Autodesk Fusion 360 part; units mm, degrees
(part 2 of 2)
sketch "All" plane through (0, 0, 0) normal (0, 0, 1) x (1, 0, 0)
  line L0 (911.9011, 0.1672) -> (886.7114, 0.1671)
  line L1 (568.1448, -296.0398) -> (568.1448, -307.8378)
  line L2 (734.5324, -64.7128) -> (810.7324, -64.7128)
  line L3 (909.9675, -283.9081) -> (916.3175, -283.9081)
  line L4 (886.7114, 0.1671) -> (886.7114, 6.5171)
  line L5 (775.9132, -250.6459) -> (775.9132, -244.2911)
  line L6 (662.6478, -251.0469) -> (662.6478, -327.2469)
  line L7 (615.7805, -143.0099) -> (615.7805, -149.3599)
  line L8 (916.3175, -296.6081) -> (909.9675, -296.6081)
  line L9 (861.3114, 6.5171) -> (861.3114, 0.1672)
  line L10 (825.1884, -118.2052) -> (825.181, -105.5052)
  line L11 (848.6114, -82.3828) -> (861.3114, -82.3828)
  line L12 (628.4805, -149.3599) -> (628.4805, -143.0099)
  line L13 (909.9675, -271.2081) -> (909.9675, -244.9009)
  line L14 (732.6938, -144.5054) -> (808.8938, -144.5054)
  line L15 (733.2164, -153.1742) -> (809.4164, -153.1742)
  line L16 (728.1176, -23.0624) -> (728.1101, -10.3624)
  line L17 (916.3175, -309.3081) -> (916.3175, -296.6081)
  line L18 (848.6114, 0.1672) -> (848.6114, 6.5171)
  line L19 (775.9132, -250.6449) -> (744.3131, -250.6449)
  line L20 (914.218, -118.2052) -> (914.2254, -105.5052)
  line L21 (874.0114, 6.5171) -> (874.0114, 0.1672)
  line L22 (561.7948, -307.8378) -> (561.7948, -320.5378)
  line L23 (916.3175, -283.9081) -> (916.3175, -271.2081)
  line L24 (653.8805, -149.3599) -> (666.5805, -149.3599)
  line L25 (817.1471, -23.0624) -> (817.1546, -10.3624)
  line L26 (825.1921, -143.6015) -> (831.6032, -143.6015)
  line L27 (809.4164, -217.5813) -> (809.4164, -232.0956)
  line L28 (732.5584, -251.0469) -> (706.9479, -251.0469)
  line L29 (831.6474, -237.2473) -> (831.6474, -220.0168)
  line L30 (788.6132, -326.8449) -> (814.2237, -326.8449)
  line L31 (827.4175, -271.2081) -> (833.7675, -271.2081)
  line L32 (810.7324, 3.1782) -> (734.4601, 2.7712)
  line L33 (886.7114, -76.0328) -> (886.7114, -82.3828)
  line L34 (628.4805, -143.0099) -> (615.7805, -143.0099)
  line L35 (831.531, -92.3716) -> (831.531, -105.5015)
  line L36 (603.0823, -149.3583) -> (615.7805, -149.3599)
  line L37 (775.9132, -333.1987) -> (788.6132, -333.1987)
  line L38 (568.3687, -250.951) -> (644.5687, -250.951)
  line L39 (568.1448, -296.0398) -> (644.3448, -296.0398)
  line L40 (561.7948, -320.5378) -> (568.1448, -320.5378)
  line L41 (861.3114, -82.3828) -> (861.3114, -76.0328)
  line L42 (706.9479, -327.2469) -> (732.5584, -327.2469)
  line L43 (815.249, -114.5749) -> (815.249, -127.2749)
  line L44 (644.5687, -287.2419) -> (568.3687, -287.2419)
  line L45 (679.2805, -231.9067) -> (666.5805, -231.9067)
  line L46 (815.249, -127.2749) -> (808.8937, -127.2749)
  line L47 (833.7675, -283.9081) -> (833.7675, -296.6081)
  line L48 (808.8938, -144.5054) -> (808.8938, -127.2749)
  line L49 (833.7675, -283.9081) -> (827.4175, -283.9081)
  line L50 (644.3448, -332.3306) -> (568.1448, -332.3306)
  line L51 (916.3175, -271.2081) -> (909.9675, -271.2081)
  line L52 (907.8032, -91.9647) -> (907.8754, -105.5015)
  line L53 (833.7675, -244.9009) -> (833.7675, -271.2081)
  line L54 (817.1546, -10.3624) -> (810.8046, -10.3587)
  line L55 (825.3026, -194.6168) -> (825.3026, -181.9168)
  line L56 (827.4175, -296.6081) -> (833.7675, -296.6081)
  line L57 (817.1434, -48.4587) -> (810.7324, -48.4587)
  line L58 (568.1448, -332.3306) -> (568.1448, -320.5378)
  line L59 (831.6032, -155.8932) -> (831.6032, -159.8556)
  line L60 (831.6474, -194.6168) -> (825.3026, -194.6168)
  line L61 (825.1921, -130.9015) -> (825.1921, -143.6015)
  line L62 (694.2479, -251.0469) -> (662.6478, -251.0469)
  line L63 (679.2805, -143.0099) -> (666.5805, -143.0099)
  line L64 (734.4601, 2.7712) -> (734.4601, -10.3587)
  line L65 (788.6132, -333.1987) -> (788.6132, -326.843)
  line L66 (907.8032, -91.9647) -> (831.531, -92.3716)
  line L67 (733.2164, -217.5813) -> (726.8664, -217.5813)
  line L68 (831.5384, -118.2015) -> (825.1884, -118.2052)
  line L69 (907.8474, -207.3168) -> (907.8474, -194.6168)
  line L70 (603.0823, -225.5583) -> (603.0823, -149.3583)
  line L71 (615.7805, -231.9067) -> (615.7805, -225.5567)
  line L72 (679.2805, -225.5567) -> (679.2805, -231.9067)
  line L73 (831.6474, -207.3168) -> (831.6474, -194.6168)
  line L74 (734.5324, -60.7504) -> (734.5324, -64.7128)
  line L75 (810.7324, 3.1782) -> (810.8046, -10.3587)
  line L76 (808.8938, -89.1749) -> (808.8938, -71.934)
  line L77 (833.7675, -309.3081) -> (827.4175, -309.3081)
  line L78 (886.7114, -76.0328) -> (911.9011, -76.0328)
  line L79 (733.2164, -192.1813) -> (726.8664, -192.1813)
  line L80 (666.5805, -225.5583) -> (653.8805, -225.5583)
  line L81 (907.8474, -229.7323) -> (907.8474, -220.0168)
  line L82 (650.9187, -275.4439) -> (650.9187, -262.7439)
  line L83 (886.7114, -82.3828) -> (874.0114, -82.3828)
  line L84 (679.2805, -149.3599) -> (679.2805, -143.0099)
  line L85 (694.2479, -251.0479) -> (694.2479, -244.6931)
  line L86 (827.4175, -309.3081) -> (827.4175, -296.6081)
  line L87 (704.6805, -149.3599) -> (704.6805, -143.0099)
  line L88 (627.6803, -165.6876) -> (615.8803, -165.6876)
  line L89 (732.6938, -136.9904) -> (732.6938, -127.2749)
  line L90 (907.8754, -105.5015) -> (907.8032, -105.5015)
  line L91 (691.9805, -231.9067) -> (691.9805, -225.5567)
  line L92 (691.9805, -143.0099) -> (691.9805, -149.3599)
  line L93 (825.2922, -207.3168) -> (825.2922, -220.0168)
  line L94 (615.8803, -185.7876) -> (627.6803, -185.7876)
  line L95 (809.4164, -217.5813) -> (815.7664, -217.5813)
  line L96 (653.8805, -231.9067) -> (641.1805, -231.9067)
  line L97 (815.7664, -204.8813) -> (809.4164, -204.8813)
  line L98 (694.2479, -333.6007) -> (706.9479, -333.6007)
  line L99 (726.8664, -179.4813) -> (733.2164, -179.4813)
  line L100 (825.2922, -220.0168) -> (831.6475, -220.0168)
  line L101 (833.7675, -309.3081) -> (833.7675, -323.8224)
  line L102 (732.6938, -101.8749) -> (726.349, -101.8749)
  line L103 (907.8474, -164.6759) -> (907.8474, -172.1909)
  line L104 (810.7324, -52.9163) -> (810.7324, -60.7504)
  line L105 (810.7324, -52.9163) -> (810.7324, -48.4587)
  line L106 (568.3687, -262.7439) -> (568.3687, -250.951)
  line L107 (726.349, -89.1749) -> (732.6938, -89.1749)
  line L108 (704.6805, -143.0099) -> (691.9805, -143.0099)
  line L109 (728.1213, -48.4587) -> (734.5324, -48.4587)
  line L110 (810.7324, -64.7128) -> (810.7324, -60.7504)
  line L111 (907.868, -118.2015) -> (907.8032, -118.2015)
  line L112 (810.7324, -35.7587) -> (810.7324, -23.0587)
  line L113 (666.5805, -231.9067) -> (666.5805, -225.5567)
  line L114 (628.4805, -225.5567) -> (628.4805, -231.9067)
  line L115 (831.6474, -181.9168) -> (831.6474, -164.6759)
  line L116 (815.7664, -192.1813) -> (815.7664, -179.4813)
  line L117 (644.3448, -296.0398) -> (644.3448, -307.8378)
  line L118 (861.3114, -76.0328) -> (874.0114, -76.0328)
  line L119 (809.4164, -232.0956) -> (733.2164, -232.0956)
  line L120 (728.1101, -10.3624) -> (734.4601, -10.3587)
  line L121 (909.9675, -323.8224) -> (909.9675, -309.3081)
  line L122 (831.6032, -159.8556) -> (907.8032, -159.8556)
  line L123 (775.9132, -326.8439) -> (775.9132, -333.1987)
  line L124 (810.7971, -23.0587) -> (810.7324, -23.0587)
  line L125 (666.5805, -143.0099) -> (666.5805, -149.3599)
  line L126 (808.8938, -71.934) -> (732.6938, -71.934)
  line L127 (823.3543, -76.0328) -> (848.6114, -76.0328)
  line L128 (909.9675, -296.6081) -> (909.9675, -283.9081)
  line L129 (825.181, -105.5052) -> (831.531, -105.5015)
  line L130 (833.7675, -323.8224) -> (909.9675, -323.8224)
  line L131 (568.1448, -307.8378) -> (561.7948, -307.8378)
  line L132 (909.9675, -244.9009) -> (833.7675, -244.9009)
  line L133 (907.8754, -105.5015) -> (907.8032, -105.5015)
  line L134 (706.9479, -244.6931) -> (706.9479, -251.0488)
  line L135 (653.8805, -143.0099) -> (641.1805, -143.0099)
  line L136 (810.7324, -35.7587) -> (817.1434, -35.7587)
  line L137 (907.8474, -237.2473) -> (831.6474, -237.2473)
  line L138 (808.8938, -101.8749) -> (815.2386, -101.8749)
  line L139 (831.6474, -164.6759) -> (907.8474, -164.6759)
  line L140 (874.0114, -82.3828) -> (874.0114, -76.0328)
  line L141 (810.7971, -23.0587) -> (817.1471, -23.0624)
  line L142 (694.2479, -244.6931) -> (706.9479, -244.6931)
  line L143 (744.3131, -326.8449) -> (775.9132, -326.8449)
  line L144 (810.8046, -10.3587) -> (810.7324, -10.3587)
  line L145 (641.1805, -143.0099) -> (641.1805, -149.3599)
  line L146 (653.8805, -149.3599) -> (653.8805, -143.0099)
  line L147 (810.8046, -10.3587) -> (810.7324, -10.3587)
  line L148 (914.2254, -105.5052) -> (907.8754, -105.5015)
  line L149 (848.6114, -76.0328) -> (848.6114, -82.3828)
  line L150 (823.3543, 0.1672) -> (823.3543, -76.0328)
  line L151 (911.9011, -76.0328) -> (911.9011, 0.1672)
  line L152 (744.3131, -250.6449) -> (744.3131, -326.8449)
  line L153 (814.2237, -326.8449) -> (814.2237, -250.6449)
  line L154 (788.6132, -244.2911) -> (788.6132, -250.6468)
  line L155 (775.9132, -244.2911) -> (788.6132, -244.2911)
  line L156 (886.7114, 6.5171) -> (874.0114, 6.5171)
  line L157 (814.2237, -250.6449) -> (788.6132, -250.6449)
  line L158 (848.6114, 6.5171) -> (861.3114, 6.5171)
  line L159 (874.0114, 0.1672) -> (861.3114, 0.1672)
  line L160 (848.6114, 0.1672) -> (823.3543, 0.1672)
  line L161 (909.9675, -309.3081) -> (916.3175, -309.3081)
  line L162 (628.4805, -149.3599) -> (641.1805, -149.3599)
  line L163 (732.5584, -327.2469) -> (732.5584, -251.0469)
  line L164 (644.5687, -275.4439) -> (650.9187, -275.4439)
  line L165 (644.3448, -307.8378) -> (650.6948, -307.8378)
  circle A0 centre (621.3303, -203.676) radius 7.75
  line L166 (728.1213, -35.7587) -> (728.1213, -48.4587)
  line L167 (627.6803, -185.7876) -> (627.6803, -165.6876)
  line L168 (815.7664, -179.4813) -> (809.4164, -179.4813)
  line L169 (717.3823, -225.5583) -> (704.6805, -225.5583)
  line L170 (615.8803, -165.6876) -> (615.8803, -185.7876)
  line L171 (815.2386, -101.8749) -> (815.2386, -89.1749)
  line L172 (732.6938, -136.9904) -> (732.6938, -144.5054)
  line L173 (808.8938, -114.5749) -> (808.8938, -101.8749)
  line L174 (914.2142, -143.6015) -> (907.8032, -143.6015)
  line L175 (831.6474, -207.3168) -> (825.2922, -207.3168)
  line L176 (653.8805, -225.5567) -> (653.8805, -231.9067)
  line L177 (641.1805, -231.9067) -> (641.1805, -225.5567)
  line L178 (615.7805, -225.5583) -> (603.0823, -225.5583)
  line L179 (733.2164, -179.4813) -> (733.2164, -153.1742)
  line L180 (650.6948, -307.8378) -> (650.6948, -320.5378)
  line L181 (831.6032, -130.9015) -> (825.1921, -130.9015)
  line L182 (732.6938, -114.5749) -> (726.3386, -114.5749)
  line L183 (726.349, -101.8749) -> (726.349, -89.1749)
  line L184 (831.6032, -143.6015) -> (831.6032, -155.8932)
  line L185 (827.4175, -283.9081) -> (827.4175, -271.2081)
  line L186 (907.8032, -148.0591) -> (907.8032, -143.6015)
  line L187 (809.4164, -153.1742) -> (809.4164, -179.4813)
  line L188 (679.2805, -149.3599) -> (691.9805, -149.3599)
  line L189 (809.4164, -192.1813) -> (815.7664, -192.1813)
  line L190 (717.3823, -149.3583) -> (717.3823, -225.5583)
  line L191 (831.5384, -118.2015) -> (831.6032, -130.9015)
  line L192 (734.5324, -48.4587) -> (734.5324, -60.7504)
  line L193 (825.3026, -181.9168) -> (831.6474, -181.9168)
  line L194 (817.1434, -35.7587) -> (817.1434, -48.4587)
  line L195 (907.8474, -200.9668) -> (907.8474, -207.3168)
  line L196 (808.8938, -114.5749) -> (815.249, -114.5749)
  line L197 (732.6938, -89.1749) -> (732.6938, -79.449)
  line L198 (732.6938, -71.934) -> (732.6938, -79.449)
  line L199 (815.2386, -89.1749) -> (808.8938, -89.1749)
  line L200 (644.5687, -287.2419) -> (644.5687, -275.4439)
  line L201 (628.4805, -231.9067) -> (615.7805, -231.9067)
  line L202 (815.7664, -217.5813) -> (815.7664, -204.8813)
  line L203 (704.6805, -231.9067) -> (691.9805, -231.9067)
  line L204 (726.8664, -192.1813) -> (726.8664, -179.4813)
  line L205 (726.3386, -127.2749) -> (732.694, -127.2749)
  line L206 (650.9187, -262.7439) -> (644.5687, -262.7439)
  line L207 (734.4676, -23.0587) -> (734.5324, -35.7587)
  line L208 (732.6938, -114.5749) -> (732.6938, -101.8749)
  line L209 (644.5687, -250.951) -> (644.5687, -262.7439)
  line L210 (907.8032, -130.9015) -> (907.8032, -118.2015)
  line L211 (733.2164, -204.8813) -> (733.2164, -192.1813)
  line L212 (914.1922, -194.6168) -> (914.1922, -181.9168)
  line L213 (706.9479, -333.6007) -> (706.9479, -327.245)
  line L214 (691.9805, -225.5583) -> (679.2805, -225.5583)
  line L215 (641.1805, -225.5583) -> (628.4805, -225.5583)
  line L216 (726.8664, -217.5813) -> (726.8664, -204.8813)
  line L217 (562.0187, -275.4439) -> (562.0187, -262.7439)
  line L218 (726.8664, -204.8813) -> (733.2164, -204.8813)
  line L219 (704.6805, -149.3599) -> (717.3823, -149.3583)
  line L220 (726.3386, -114.5749) -> (726.3386, -127.2749)
  line L221 (734.5324, -35.7587) -> (728.1213, -35.7587)
  line L222 (732.6938, -108.2249) -> (732.6938, -114.5749)
  line L223 (809.4164, -192.1813) -> (809.4164, -204.8813)
  line L224 (733.2164, -232.0956) -> (733.2164, -217.5813)
  line L225 (734.4676, -23.0587) -> (728.1176, -23.0624)
  line L226 (810.7324, -23.0587) -> (810.7971, -23.0587)
  line L227 (907.8474, -229.7323) -> (907.8474, -237.2473)
  line L228 (568.3687, -275.4439) -> (562.0187, -275.4439)
  line L229 (907.8474, -181.9168) -> (907.8474, -172.1909)
  line L230 (694.2479, -327.2459) -> (694.2479, -333.6007)
  line L231 (562.0187, -262.7439) -> (568.3687, -262.7439)
  line L232 (907.8032, -118.2015) -> (907.868, -118.2015)
  line L233 (907.8032, -130.9015) -> (914.2142, -130.9015)
  line L234 (907.868, -118.2015) -> (914.218, -118.2052)
  line L235 (907.8474, -207.3168) -> (914.2026, -207.3168)
  line L236 (907.8474, -194.6168) -> (914.1922, -194.6168)
  line L237 (914.2142, -130.9015) -> (914.2142, -143.6015)
  line L238 (914.1922, -181.9168) -> (907.8474, -181.9168)
  line L239 (907.8032, -159.8556) -> (907.8032, -155.8932)
  line L240 (914.2026, -220.0168) -> (907.8473, -220.0168)
  line L241 (914.2026, -207.3168) -> (914.2026, -220.0168)
  line L242 (650.6948, -320.5378) -> (644.3448, -320.5378)
  line L243 (644.3448, -320.5378) -> (644.3448, -332.3306)
  line L244 (662.6478, -327.2469) -> (694.2479, -327.2469)
  line L245 (704.6805, -225.5567) -> (704.6805, -231.9067)
  line L246 (907.8032, -148.0591) -> (907.8032, -155.8932)
  line L247 (568.3687, -287.2419) -> (568.3687, -275.4439)
  line L248 (397.5742, -236.0352) -> (406.5544, -245.0155)
  line L249 (573.5153, -137.8573) -> (560.1063, -137.857)
  line L250 (363.4063, -203.0135) -> (363.4063, -198.5559)
  line L251 (557.4213, -236.0789) -> (548.441, -245.0591)
  line L252 (369.8167, -198.5559) -> (363.4063, -198.5559)
  line L253 (470.8992, -334.3082) -> (483.5992, -334.3082)
  line L254 (458.506, -174.1353) -> (458.506, -180.4853)
  line L255 (463.6102, -251.8234) -> (463.6102, -270.8934)
  line L256 (421.517, -137.8428) -> (407.7058, -137.8438)
  line L257 (470.8992, -334.3082) -> (470.8992, -327.9582)
  line L258 (363.4779, -160.4559) -> (363.4063, -160.4559)
  line L259 (561.9151, -240.5727) -> (557.4213, -236.0789)
  line L260 (420.101, -307.0939) -> (413.751, -307.0939)
  line L261 (420.101, -319.7939) -> (420.101, -307.0939)
  line L262 (433.3163, -149.6424) -> (433.3163, -162.3424)
  line L263 (369.8205, -173.1597) -> (369.8279, -160.4597)
  line L264 (363.4063, -185.8559) -> (363.4063, -173.1559)
  line L265 (458.506, -180.4853) -> (471.206, -180.4853)
  line L266 (395.0058, -137.8447) -> (381.5778, -137.8457)
  line L267 (566.4089, -227.1059) -> (575.3891, -218.1257)
  line L268 (388.5939, -227.055) -> (379.6136, -218.0747)
  line L269 (388.5939, -236.0352) -> (393.084, -240.5253)
  line L270 (471.206, -174.1353) -> (483.906, -174.1353)
  line L271 (421.517, -137.8428) -> (439.6663, -137.8444)
  line L272 (379.6136, -218.0747) -> (375.1235, -222.5648)
  line L273 (363.4705, -173.1559) -> (363.4063, -173.1559)
  line L274 (457.8096, -174.1353) -> (458.506, -174.1353)
  line L275 (413.751, -334.3082) -> (428.2616, -334.3082)
  line L276 (540.751, -294.3939) -> (534.401, -294.3939)
  line L277 (570.8953, -231.5924) -> (566.4089, -227.1059)
  line L278 (515.351, -174.1353) -> (497.3025, -174.1353)
  line L279 (363.405, -137.8457) -> (381.5778, -137.8457)
  line L280 (368.4332, -215.8745) -> (375.1235, -222.5648)
  line L281 (521.7957, -149.6424) -> (521.7958, -162.3424)
  line L282 (363.4705, -173.1559) -> (369.8205, -173.1597)
  line L283 (540.751, -261.7367) -> (540.751, -269.2517)
  line L284 (363.4063, -203.0135) -> (363.4063, -210.8477)
  line L285 (363.4063, -210.8477) -> (368.4332, -215.8745)
  line L286 (591.8598, -137.8621) -> (573.5095, -137.8621)
  line L287 (561.9151, -240.5727) -> (570.8953, -231.5924)
  line L288 (515.5406, -137.7622) -> (515.4787, -149.6424)
  line L289 (420.101, -294.3939) -> (420.101, -281.6939)
  line L290 (496.606, -174.1353) -> (496.606, -180.4853)
  line L291 (384.1038, -231.5451) -> (393.084, -240.5253)
  line L292 (384.1038, -231.5451) -> (388.5939, -227.055)
  line L293 (496.2992, -334.3082) -> (508.9992, -334.3082)
  line L294 (592.0667, -185.7991) -> (585.7167, -185.7991)
  line L295 (592.0667, -202.906) -> (592.0667, -210.421)
  line L296 (579.8756, -222.6121) -> (586.7528, -215.7349)
  line L297 (515.4457, -149.6424) -> (521.7957, -149.6424)
  line L298 (592.0667, -210.421) -> (586.7528, -215.7349)
  line L299 (560.1063, -137.857) -> (560.1063, -144.1995)
  line L300 (420.101, -307.0939) -> (413.751, -307.0939)
  line L301 (591.8598, -155.9924) -> (591.8598, -137.8621)
  line L302 (521.6992, -327.9582) -> (508.9992, -327.9582)
  line L303 (369.8167, -185.8559) -> (369.8167, -198.5559)
  line L304 (540.751, -281.6939) -> (540.751, -269.2517)
  line L305 (420.101, -281.6939) -> (413.751, -281.6939)
  line L306 (433.3163, -162.3424) -> (439.6663, -162.3424)
  line L307 (363.4063, -160.4559) -> (363.4063, -155.9924)
  line L308 (592.0667, -137.8621) -> (592.0667, -155.9924)
  line L309 (496.606, -174.1353) -> (497.3025, -174.1353)
  line L310 (439.6663, -137.8444) -> (439.6663, -149.6424)
  line L311 (526.2367, -334.3082) -> (540.751, -334.3082)
  line L312 (508.9992, -327.9582) -> (508.9992, -334.3082)
  line L313 (547.4063, -137.8568) -> (533.5887, -137.8566)
  line L314 (439.6657, -162.3424) -> (439.6646, -174.1353)
  line L315 (521.6992, -334.3082) -> (521.6992, -327.9582)
  line L316 (420.101, -319.7939) -> (420.101, -307.0939)
  line L317 (491.4202, -270.8934) -> (491.4202, -251.8234)
  line L318 (445.4992, -327.9582) -> (432.7992, -327.9582)
  line L319 (483.5992, -327.9582) -> (483.5992, -334.3082)
  line L320 (478.8502, -270.8934) -> (491.4202, -270.8934)
  line L321 (521.6992, -334.3082) -> (526.2367, -334.3082)
  line L322 (463.6102, -270.8934) -> (476.1802, -270.8934)
  line L323 (395.0058, -137.8447) -> (395.0058, -144.1995)
  line L324 (573.5095, -137.8621) -> (573.5153, -137.8573)
  line L325 (439.6646, -174.1353) -> (457.8096, -174.1353)
  line L326 (420.101, -319.7939) -> (420.101, -307.0939)
  line L327 (478.8502, -251.8234) -> (478.8502, -270.8934)
  line L328 (476.1802, -270.8934) -> (476.1802, -251.8234)
  line L329 (420.101, -307.0939) -> (413.751, -307.0939)
  line L330 (496.606, -180.4853) -> (483.906, -180.4853)
  line L331 (491.4202, -251.8234) -> (478.8502, -251.8234)
  line L332 (592.0667, -179.4491) -> (592.0667, -173.0991)
  line L333 (496.2992, -334.3082) -> (496.2992, -327.9582)
  line L334 (445.4992, -334.3082) -> (445.4992, -327.9582)
  line L335 (592.0667, -155.9924) -> (591.8598, -155.9924)
  line L336 (395.0058, -144.1995) -> (407.7058, -144.1995)
  line L337 (420.101, -281.6939) -> (413.8811, -281.6939)
  line L338 (515.351, -174.1353) -> (515.4458, -162.3424)
  line L339 (408.7815, -256.2228) -> (413.9171, -261.3584)
  line L340 (546.0649, -256.4228) -> (552.9348, -249.5529)
  line L341 (483.906, -180.4853) -> (483.906, -174.1353)
  line L342 (432.7992, -327.9582) -> (432.7992, -334.3082)
  line L343 (471.206, -180.4853) -> (471.206, -174.1353)
  line L344 (540.751, -334.3082) -> (540.751, -319.7939)
  line L345 (413.9171, -269.1441) -> (413.8811, -281.6939)
  line L346 (534.401, -281.6939) -> (540.751, -281.6939)
  line L347 (533.5887, -137.8566) -> (515.5406, -137.7622)
  line L348 (591.8655, -137.8573) -> (591.8598, -137.8621)
  line L349 (560.1063, -144.1995) -> (547.4063, -144.1995)
  line L350 (534.401, -307.0939) -> (540.751, -307.0939)
  line L351 (413.751, -294.3939) -> (420.101, -294.3939)
  line L352 (439.6663, -149.6424) -> (433.3163, -149.6424)
  line L353 (432.7992, -334.3082) -> (428.2616, -334.3082)
  line L354 (496.2992, -327.9582) -> (483.5992, -327.9582)
  line L355 (413.9171, -261.3584) -> (413.9171, -269.1441)
  line L356 (534.401, -319.7939) -> (534.401, -307.0939)
  line L357 (413.751, -294.3939) -> (420.101, -294.3939)
  line L358 (445.4992, -334.3082) -> (458.1992, -334.3082)
  line L359 (413.751, -294.3939) -> (413.751, -307.0939)
  line L360 (458.1992, -327.9582) -> (458.1992, -334.3082)
  line L361 (591.8598, -137.8621) -> (592.0667, -137.8621)
  line L362 (420.101, -319.7939) -> (413.7474, -319.7939)
  line L363 (592.0667, -160.3991) -> (592.0667, -155.9924)
  line L364 (402.0643, -249.5056) -> (408.7815, -256.2228)
  line L365 (406.5544, -245.0155) -> (402.0643, -249.5056)
  line L366 (420.101, -294.3939) -> (420.101, -281.6939)
  line L367 (592.0667, -185.7991) -> (592.0667, -173.0991)
  line L368 (585.7167, -173.0991) -> (585.7167, -160.3991)
  line L369 (573.5153, -137.8573) -> (591.8655, -137.8573)
  line L370 (420.101, -307.0939) -> (413.751, -307.0939)
  line L371 (592.0667, -202.906) -> (592.0667, -198.4991)
  line L372 (420.101, -319.7939) -> (420.101, -307.0939)
  line L373 (420.101, -294.3939) -> (420.101, -281.6939)
  line L374 (413.7474, -319.7939) -> (413.751, -334.3082)
  line L375 (592.0667, -173.0991) -> (585.7167, -173.0991)
  line L376 (585.7167, -185.7991) -> (585.7167, -198.4991)
  line L377 (413.751, -294.3939) -> (420.101, -294.3939)
  line L378 (547.4063, -144.1995) -> (547.4063, -137.8568)
  line L379 (585.7167, -198.4991) -> (592.0667, -198.4991)
  line L380 (585.7167, -160.3991) -> (592.0667, -160.3991)
  line L381 (521.7958, -162.3424) -> (515.4458, -162.3424)
  circle A1 centre (550.3615, -182.856) radius 4.83
  line L382 (363.4063, -185.8559) -> (369.8167, -185.8559)
  line L383 (420.101, -281.6939) -> (413.751, -281.6939)
  line L384 (369.8279, -160.4597) -> (363.4779, -160.4559)
  line L385 (548.441, -245.0591) -> (552.9349, -249.553)
  line L386 (575.3891, -218.1257) -> (579.8756, -222.6121)
  line L387 (470.8992, -327.9582) -> (458.1992, -327.9582)
  line L388 (540.751, -319.7939) -> (534.401, -319.7939)
  line L389 (540.751, -307.0939) -> (540.751, -294.3939)
  line L390 (476.1802, -251.8234) -> (463.6102, -251.8234)
  line L391 (566.4052, -236.0825) -> (561.9151, -240.5727)
  line L392 (407.7058, -144.1995) -> (407.7058, -137.8438)
  line L393 (363.4063, -155.9924) -> (363.405, -137.8457)
  line L394 (546.0649, -256.4228) -> (540.751, -261.7367)
  line L395 (534.401, -294.3939) -> (534.401, -281.6939)
  line L396 (393.084, -240.5253) -> (397.5742, -236.0352)
  line L397 (-272.5268, 143.985) -> (-272.5268, 143.985)
  line L398 (-272.5268, 125.8421) -> (-272.5268, 125.8421)
  line L399 (-272.5268, 125.8421) -> (-272.5268, 125.8421)
  line L400 (-254.3839, 125.8421) -> (-254.3839, 125.8421)
  line L401 (572.9189, 65.7657) -> (585.6189, 65.7657)
  line L402 (655.4671, 72.1157) -> (640.9565, 72.1157)
  line L403 (560.2189, 65.7657) -> (560.2189, 72.1157)
  line L404 (528.4671, 19.5014) -> (528.4671, 7.0592)
  line L405 (610.7121, -88.0572) -> (610.7121, -81.7072)
  line L406 (483.5014, -76.3934) -> (483.5014, -63.6934)
  line L407 (598.3189, 65.7657) -> (611.0189, 65.7657)
  line L408 (610.7121, -81.7072) -> (598.0121, -81.7072)
  line L409 (547.5189, 72.1157) -> (542.9814, 72.1157)
  line L410 (528.4671, -0.4558) -> (528.4671, 7.0592)
  line L411 (502.8129, -26.11) -> (507.303, -21.6198)
  line L412 (572.9189, 72.1157) -> (572.9189, 65.7657)
  line L413 (412.5367, -266.5161) -> (412.5367, -266.5161)
  line L414 (629.5524, -99.8501) -> (629.5535, -88.0572)
  line L415 (635.9018, -112.5501) -> (635.9018, -99.8501)
  line L416 (520.7771, -17.1334) -> (516.2832, -12.6395)
  line L417 (647.7011, -124.3497) -> (629.5518, -124.3481)
  line L418 (493.829, -44.0668) -> (489.3425, -39.5804)
  line L419 (523.1532, -5.7697) -> (516.2833, -12.6396)
  line L420 (623.7189, 72.1157) -> (611.0189, 72.1157)
  line L421 (598.3189, 72.1157) -> (598.3189, 65.7657)
  line L422 (483.5014, -101.7934) -> (477.1514, -101.7934)
  line L423 (483.5014, -89.0934) -> (483.5014, -101.7934)
  line L424 (477.1514, -82.7434) -> (477.1514, -89.0934)
  line L425 (509.1118, -117.9929) -> (521.8118, -117.9929)
  line L426 (598.0121, -81.7072) -> (598.0121, -88.0572)
  line L427 (483.5014, -63.6934) -> (477.1514, -63.6934)
  line L428 (636.4189, 72.1157) -> (640.9565, 72.1157)
  line L429 (553.6775, -124.437) -> (553.7394, -112.5501)
  line L430 (542.9814, 72.1157) -> (528.4671, 72.1157)
  line L431 (623.7189, 72.1157) -> (623.7189, 65.7657)
  line L432 (572.6121, -88.0572) -> (572.6121, -81.7072)
  line L433 (572.6121, -81.7072) -> (585.3121, -81.7072)
  line L434 (547.5189, 65.7657) -> (560.2189, 65.7657)
  line L435 (629.5535, -88.0572) -> (611.4085, -88.0572)
  line L436 (572.6121, -88.0572) -> (571.9156, -88.0572)
  line L437 (394.3938, -266.5161) -> (394.3938, -266.5161)
  line L438 (611.0189, 65.7657) -> (611.0189, 72.1157)
  line L439 (629.5518, -112.5501) -> (635.9018, -112.5501)
  line L440 (636.4189, 65.7657) -> (636.4189, 72.1157)
  line L441 (585.6189, 65.7657) -> (585.6189, 72.1157)
  line L442 (509.1118, -124.3429) -> (509.1118, -117.9929)
  line L443 (611.4085, -88.0572) -> (610.7121, -88.0572)
  line L444 (528.4671, 57.6014) -> (534.8171, 57.6014)
  line L445 (553.7724, -112.5501) -> (547.4224, -112.5501)
  line L446 (547.4223, -99.8501) -> (553.7723, -99.8501)
  line L447 (528.4671, 72.1157) -> (528.4671, 57.6014)
  line L448 (535.6294, -124.3429) -> (553.6775, -124.437)
  line L449 (477.1514, -59.2865) -> (477.1514, -51.7715)
  line L450 (394.3938, -266.5161) -> (394.3938, -266.5161)
  line L451 (521.8118, -117.9929) -> (521.8118, -124.3429)
  line L452 (553.8671, -88.0572) -> (571.9156, -88.0572)
  line L453 (528.4671, 32.2014) -> (534.8171, 32.2014)
  line L454 (511.7969, -26.1136) -> (520.7771, -17.1334)
  line L455 (477.1514, -89.0934) -> (483.5014, -89.0934)
  line L456 (635.9018, -99.8501) -> (629.5518, -99.8501)
  line L457 (534.8171, 44.9014) -> (528.4671, 44.9014)
  line L458 (572.9189, 72.1157) -> (560.2189, 72.1157)
  line L459 (394.3938, -248.3733) -> (394.3938, -248.3733)
  line L460 (477.1514, -59.2865) -> (477.1514, -63.6934)
  line L461 (521.8118, -124.3429) -> (535.6294, -124.3429)
  line L462 (489.3425, -39.5804) -> (482.4653, -46.4576)
  line L463 (585.3121, -81.7072) -> (585.3121, -88.0572)
  line L464 (547.4224, -112.5501) -> (547.4223, -99.8501)
  line L465 (623.7189, 65.7657) -> (636.4189, 65.7657)
  line L466 (523.1532, -5.7697) -> (528.4671, -0.4558)
  line L467 (534.8171, 57.6014) -> (534.8171, 44.9014)
  line L468 (553.8671, -88.0572) -> (553.7723, -99.8501)
  line L469 (498.3228, -30.6001) -> (502.8092, -35.0866)
  line L470 (507.303, -21.6198) -> (498.3228, -30.6001)
  line L471 (547.5189, 72.1157) -> (547.5189, 65.7657)
  line L472 (507.303, -21.6198) -> (511.7969, -26.1136)
  line L473 (534.8171, 19.5014) -> (528.4671, 19.5014)
  line L474 (528.4671, 44.9014) -> (528.4671, 32.2014)
  line L475 (629.5518, -124.3481) -> (629.5518, -112.5501)
  line L476 (477.1514, -76.3934) -> (483.5014, -76.3934)
  line L477 (477.1514, -76.3934) -> (477.1514, -89.0934)
  line L478 (477.1514, -51.7715) -> (482.4653, -46.4576)
  line L479 (534.8171, 32.2014) -> (534.8171, 19.5014)
  line L480 (598.0121, -88.0572) -> (585.3121, -88.0572)
  line L481 (598.3189, 72.1157) -> (585.6189, 72.1157)
  line L482 (502.8092, -35.0866) -> (493.829, -44.0668)
  line L483 (655.4708, 57.6014) -> (655.4671, 72.1157)
  line L484 (705.8118, -59.1789) -> (705.8118, -51.3448)
  line L485 (705.7477, -89.0366) -> (705.8118, -89.0366)
  line L486 (700.7849, -46.318) -> (694.0946, -39.6277)
  line L487 (655.4671, 32.2014) -> (649.1171, 32.2014)
  line L488 (674.2123, -117.9929) -> (661.5123, -117.9929)
  line L489 (705.8118, -106.2001) -> (705.8131, -124.3468)
  line L490 (661.5123, -117.9929) -> (661.5123, -124.3487)
  line L491 (674.2123, -124.3478) -> (674.2123, -117.9929)
  line L492 (699.4014, -63.6366) -> (705.8118, -63.6366)
  line L493 (705.8118, -51.3448) -> (700.7849, -46.318)
  line L494 (685.1143, -30.6474) -> (680.6242, -35.1375)
  line L495 (705.7477, -89.0366) -> (699.3977, -89.0328)
  line L496 (699.3977, -89.0328) -> (699.3902, -101.7328)
  line L497 (674.2123, -124.3478) -> (687.6403, -124.3468)
  line L498 (649.1171, 57.6014) -> (649.1171, 44.9014)
  line L499 (705.8118, -59.1789) -> (705.8118, -63.6366)
  line L500 (680.6242, -26.1573) -> (676.1341, -21.6672)
  line L501 (680.6242, -35.1375) -> (689.6045, -44.1178)
  line L502 (705.7402, -101.7366) -> (705.8118, -101.7366)
  line L503 (649.1171, 44.9014) -> (655.4671, 44.9014)
  line L504 (649.1171, 19.5014) -> (655.4671, 19.5014)
  line L505 (649.1171, 57.6014) -> (649.1171, 44.9014)
  line L506 (655.4671, 32.2014) -> (649.1171, 32.2014)
  line L507 (705.8131, -124.3468) -> (687.6403, -124.3468)
  line L508 (667.1538, -12.6869) -> (660.4366, -5.9697)
  line L509 (699.3902, -101.7328) -> (705.7402, -101.7366)
  line L510 (649.1171, 19.5014) -> (655.4671, 19.5014)
  line L511 (655.4671, 32.2014) -> (655.4671, 44.9014)
  line L512 (649.1171, 32.2014) -> (649.1171, 19.5014)
  line L513 (699.4014, -76.3366) -> (699.4014, -63.6366)
  line L514 (685.1143, -30.6474) -> (676.1341, -21.6672)
  line L515 (671.644, -26.1573) -> (662.6637, -17.177)
  line L516 (660.4366, -5.9697) -> (655.301, -0.8341)
  line L517 (647.7011, -124.3497) -> (661.5123, -124.3487)
  line L518 (655.4671, 32.2014) -> (649.1171, 32.2014)
  line L519 (649.1171, 44.9014) -> (655.4671, 44.9014)
  line L520 (655.301, -0.8341) -> (655.301, 6.9516)
  line L521 (689.6045, -44.1178) -> (694.0946, -39.6277)
  line L522 (649.1171, 44.9014) -> (655.4671, 44.9014)
  line L523 (676.1341, -21.6672) -> (671.644, -26.1573)
  line L524 (705.8118, -76.3366) -> (699.4014, -76.3366)
  line L525 (705.8118, -101.7366) -> (705.8118, -106.2001)
  line L526 (649.1171, 44.9014) -> (655.4671, 44.9014)
  line L527 (649.1171, 57.6014) -> (649.1171, 44.9014)
  line L528 (655.301, 6.9516) -> (655.337, 19.5014)
  line L529 (649.1171, 32.2014) -> (649.1171, 19.5014)
  line L530 (705.8118, -76.3366) -> (705.8118, -89.0366)
  line L531 (662.6637, -17.177) -> (667.1538, -12.6869)
  line L532 (649.1171, 32.2014) -> (649.1171, 19.5014)
  line L533 (649.1171, 19.5014) -> (655.337, 19.5014)
  line L534 (649.1171, 57.6014) -> (649.1171, 44.9014)
  line L535 (649.1171, 57.6014) -> (655.4708, 57.6014)
  line L536 (477.1514, -124.3429) -> (509.1118, -124.3429)
  line L537 (477.1514, -124.3429) -> (477.1514, -101.7934)
  point P0 (556.8337, -356.5257)
  point P1 (413.751, -334.3082)
  point P2 (413.751, -334.3082)
  dimension "d164" = 76.2
  dimension "d165" = 76.2
  dimension "d166" = 76.2
  dimension "d167" = 76.2
  dimension "d168" = 76.2
  dimension "d169" = 76.2
  dimension "d170" = 76.2
  dimension "d171" = 76.2
  dimension "d172" = 3.9624
  dimension "d173" = 3.9624
  dimension "d174" = 11.8
  dimension "d175" = 20.1
  dimension "d176" = 15.5
  dimension "d179" = 6.35
  dimension "d180" = 12.7
  dimension "d181" = 9.66
  dimension "d182" = 12.57
  dimension "d183" = 19.07
  dimension "d184" = 12.57
  dimension "d185" = 19.07
  dimension "d188" = 6.35
  dimension "d189" = 12.7
  constraint vertical L186
  constraint horizontal L233
  constraint vertical L237
  constraint horizontal L174
  constraint coincident L90.end L186
  constraint perpendicular L133 L186
  constraint perpendicular L111 L186
  constraint collinear L186 L210
  constraint perpendicular L174 L246
  constraint horizontal L244
  constraint vertical L163
  constraint horizontal L28
  constraint vertical L6
  constraint coincident L244.end L230
  constraint coincident L42.start L213
  constraint collinear L42 L244
  constraint vertical L1
  constraint horizontal L131
  constraint vertical L22
  constraint horizontal L40
  constraint horizontal L39
  constraint vertical L117
  constraint horizontal L50
  constraint vertical L58
  constraint horizontal L143
  constraint vertical L153
  constraint horizontal L157
  constraint vertical L152
  constraint coincident L143.end L123
  constraint coincident L30.start L65
  constraint collinear L30 L143
  constraint horizontal L127
  constraint vertical L151
  constraint horizontal L0
  constraint vertical L150
  constraint collinear L118 L127
  constraint coincident L78.start L33
  constraint collinear L78 L118
  constraint horizontal L15
  constraint vertical L187
  constraint horizontal L119
  constraint vertical L224
  constraint collinear L179 L224
  constraint collinear L211 L224
  constraint coincident L107.end L89
  constraint parallel L197 L198
  constraint parallel L89 L172
  constraint perpendicular L14 L172
  constraint perpendicular L14 L48
  constraint perpendicular L126 L198
  constraint symmetric L121.start L130.end L130
  constraint symmetric L101.end L130.start L130
  constraint vertical L190
  constraint horizontal L169
  constraint vertical L70
  constraint collinear L29 L115
  constraint coincident L29.end L100
  constraint collinear L29 L73
  constraint collinear L53 L101
  constraint collinear L47 L53
  constraint perpendicular L52 L66
  constraint vertical L35
  constraint coincident L215.end L114
  constraint coincident L178.start L71
  constraint collinear L169 L178
  constraint coincident L80.end L176
  constraint coincident L215.start L177
  constraint collinear L169 L215
  constraint coincident L214.end L72
  constraint coincident L80.start L113
  constraint collinear L80 L169
  constraint coincident L169.end L245
  constraint coincident L214.start L91
  constraint collinear L169 L214
  constraint collinear L27 L187
  constraint collinear L187 L223
  constraint collinear L48 L76
  constraint coincident L48.end L46
  constraint collinear L48 L173
  constraint coincident L28.end L134
  constraint coincident L62.start L85
  constraint collinear L28 L62
  constraint collinear L0 L160
  constraint collinear L0 L159
  constraint coincident L157.end L154
  constraint coincident L19.start L5
  constraint collinear L19 L157
  constraint collinear L117 L243
  constraint collinear L106 L247
  constraint parallel L59 L184
  constraint perpendicular L122 L246
  constraint perpendicular L122 L239
  constraint vertical L105
  constraint horizontal L136
  constraint vertical L194
  constraint horizontal L57
  constraint coincident L144.end L105
  constraint perpendicular L105 L144
  constraint perpendicular L105 L124
  constraint collinear L105 L112
  constraint perpendicular L57 L104
  constraint perpendicular L32 L75
  constraint vertical L64
  constraint parallel L74 L192
  constraint perpendicular L2 L104
  constraint perpendicular L2 L110
  constraint vertical L250
  constraint coincident L296.start L340
  constraint collinear L249 L313
  constraint collinear L274 L309
  constraint collinear L270 L274
  constraint collinear L256 L266
  constraint horizontal L382
  constraint vertical L303
  constraint horizontal L252
  constraint coincident L258.end L250
  constraint perpendicular L250 L258
  constraint perpendicular L250 L273
  constraint collinear L250 L307
  constraint collinear L250 L264
  constraint parallel L269 L280
  constraint perpendicular L269 L396
  constraint perpendicular L248 L396
  constraint coincident L364.start L280
  constraint perpendicular L280 L365
  constraint collinear L280 L291
  constraint collinear L291 L364
  constraint horizontal L325
  constraint horizontal L278
  constraint perpendicular L271 L314
  constraint vertical L310
  constraint perpendicular L266 L393
  constraint horizontal L279
  constraint horizontal L369
  constraint horizontal L286
  constraint vertical L301
  constraint vertical L308
  constraint perpendicular L252 L284
  constraint parallel L280 L285
  constraint parallel L339 L364
  constraint vertical L355
  constraint parallel L295 L371
  constraint parallel L296 L298
  constraint parallel L340 L394
  constraint parallel L283 L304
  constraint coincident P2 P1
  constraint parallel L275 L353
  constraint parallel L311 L388
  constraint perpendicular L344 L388
  constraint horizontal L352
  constraint vertical L262
  constraint horizontal L306
  constraint coincident L314.start L306
  constraint coincident L288.end L297
  constraint horizontal L322
  constraint vertical L328
  constraint horizontal L390
  constraint vertical L255
  constraint horizontal L320
  constraint vertical L317
  constraint horizontal L331
  constraint vertical L327
  constraint coincident L418.end L419
  constraint collinear L436 L443
  constraint collinear L443 L480
  constraint collinear L497 L517
  constraint coincident L502.end L499
  constraint perpendicular L499 L502
  constraint perpendicular L485 L499
  constraint collinear L499 L525
  constraint collinear L499 L530
  constraint parallel L486 L500
  constraint perpendicular L500 L523
  constraint perpendicular L515 L523
  constraint coincident L508.start L486
  constraint perpendicular L486 L531
  constraint collinear L486 L514
  constraint collinear L508 L514
  constraint perpendicular L414 L417
  constraint perpendicular L489 L497
  constraint perpendicular L484 L492
  constraint parallel L486 L493
  constraint parallel L508 L516
  constraint parallel L449 L460
  constraint parallel L462 L478
  constraint parallel L419 L466
  constraint parallel L404 L410
  constraint parallel L402 L428
  constraint parallel L430 L444
  constraint perpendicular L444 L447
  constraint coincident L414.start L456
  constraint coincident L429.end L445
  measures "d164" distance of L6.end L6.start
  measures "d165" distance of L39.end L1.start
  measures "d166" distance of L44.start L44.end
  measures "d167" distance of L19.end L143.start
  measures "d168" distance of L150.start L127.start
  measures "d169" distance of L15.start L15.end
  measures "d170" distance of L14.start L14.end
  measures "d171" distance of L36.start L70.start
  measures "d172" distance of L59.end L59.start
  measures "d173" distance of L74.start L2.start
  measures "d174" distance of L88.start L88.end
  measures "d175" distance of L88.start L94.end
  measures "d176" diameter of A0
  measures "d179" distance of L269.end L248.start
  measures "d180" distance of L248.start L248.end
  measures "d181" diameter of A1
  measures "d182" distance of L255.end L322.end
  measures "d183" distance of L255.end L255.start
  measures "d184" distance of L320.start L317.start
  measures "d185" distance of L327.start L320.start
  measures "d188" distance of L500.end L515.start
  measures "d189" distance of L515.end L515.start
component "Bottom" placed x (1, 0, 0) y (0, 1, 0) z (0, 0, 1) at (0, 0, 0)
component "Top" placed x (1, 0, 0) y (0, 1, 0) z (0, 0, 1) at (-254, 0, 82.5468)
component "Wall1" placed x (0, 0, -1) y (0, 1, 0) z (1, 0, 0) at (120.65, -337.0777, 307.8265)
component "Wall2" placed x (0, 0, 1) y (0.707107, 0.707107, 0) z (-0.707107, 0.707107, 0) at (-173.2892, -227.7105, -218.3988)
component "Wall4" placed x (-1, 0, 0) y (0, 0, 1) z (0, 1, 0) at (933.3098, 187.5744, -233.0666)
component "Wall5" placed x (0, 0, -1) y (-0.000001, 1, 0) z (1, 0.000001, 0) at (99.1607, 79.1027, 757.1027)
component "Wall6" placed x (1, 0, 0) y (0, 0, 1) z (0, -1, 0) at (-637.0591, 162.7071, -223.4293)
component "Wall7" placed x (1, 0, 0) y (0, 0, 1) z (0, -1, 0) at (-727.8708, 198.9928, -126.0126)
component "Wall8" placed x (0, 0, 1) y (0, -1, 0) z (1, 0, 0) at (17.0311, 232.4349, -667.9789)
component "Wall9" placed x (0, 0, -1) y (-0.000586, -1, 0) z (-1, 0.000586, 0) at (-43.6179, 694.5593, 67.9073)
component "Wall10" placed x (0, 0, -1) y (-0.707107, 0.707107, 0) z (0.707107, 0.707107, 0) at (302.4804, -229.3645, 67.8815)
component "Wall11" placed x (0, 0, -1) y (0, 1, 0) z (1, 0, 0) at (0, -340.4938, 70.0068)
component "Wall12" placed x (1, 0, 0) y (0, 0, -1) z (0, 1, 0) at (-78.8178, 0, 359.41)
component "Wall3 (1)" placed x (0, 0, 1) y (0, -1, 0) z (1, 0, 0) at (171.9658, 694.62, -220.1814)
component "Wall3" placed x (1, 0, 0) y (0, 1, 0) z (0, 0, 1) at (0, 0, 0) in component "Wall3 (1)"
named bodies: "Wall12", "Wall1", "Wall10", "Wall11", "Wall5", "Wall8", "Wall7", "Wall6", "Wall2", "Wall9", "Wall4"
